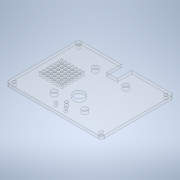
# Autodesk Inventor part: x_axis_plate_top_t
Saved by Autodesk Inventor 2022 (Build 260153000, 153)
## iProperties
Created: 2021-04-16
Part Number: x_axis_plate_top_t
Material: PET Plastic
Document SubType Name: Modeling
Designer: Fabijan_Sven
Density: 1.541 g/cm^3
Appearance: Polycarbonate - Clear
Mass: 164.884 g
Surface Area: 477.118 cm^2
Volume: 106.998 cm^3
Author: Fabijan_Sven
Autodesk Inventor part; units mm, degrees
ref_plane "YZ Plane" through (0, 0, 0) normal (1, 0, 0) x (0, 1, 0)
ref_plane "XZ Plane" through (0, 0, 0) normal (0, 1, 0) x (-1, 0, 0)
ref_plane "XY Plane" through (0, 0, 0) normal (0, 0, 1) x (1, 0, 0)
sketch "Sketch1" plane through (0, 0, 0) normal (0, 1, 0) x (-1, 0, 0)
  line L0 (-81, 62) -> (81, 62)
  line L1 (81, 62) -> (81, -62)
  line L2 (81, -62) -> (-81, -62)
  line L3 (-81, -62) -> (-81, 62)
  point P0 (0, 0)
  dimension "d117" = 124
  dimension "d118" = 162
  dimension "d119" = 81
  dimension "d120" = 62
  constraints: 8 end point, 2 parallel, 1 horizontal, 1 perpendicular
  measures "d117" distance between parallel lines of L2 L0
  measures "d118" distance between parallel lines of L1 L3
  measures "d119" distance from line of point (0, 0) L1
  measures "d120" distance from line of L2 point (0, 0)
extrude "Extrusion1" add sketch "Sketch1" along normal blind 5
fillet "Fillet1" radius 5 4 edges at (81, 2.5, 62) (81, 2.5, -62) (-81, 2.5, -62) (-81, 2.5, 62)
sketch "Sketch3" plane through (0, 5, 0) normal (0, 1, 0) x (1, 0, 0)
  circle A0 centre (74, -55) radius 3
  circle A1 centre (-74, -55) radius 3
  circle A2 centre (-74, 55) radius 3
  circle A3 centre (74, 55) radius 3
  line L0 (-76, -62) -> (76, -62) projected
  line L1 (81, -57) -> (81, 57) projected
  line L2 (-81, 57) -> (-81, -57) projected
  line L3 (76, 62) -> (-76, 62) projected
  point P0 (0, 0)
  dimension "d121" = 6
  dimension "d122" = 7
  dimension "d123" = 7
  dimension "d124" = 7
  dimension "d125" = 7
  constraints: 4 centre point, 3 equal radius, 2 horizontal alignment, 2 vertical alignment
  measures "d121" diameter of A0
  measures "d122" distance from line of L0 A0.centre
  measures "d123" distance from line of L1 A0.centre
  measures "d124" distance from line of L2 A1.centre
  measures "d125" distance from line of L3 A3.centre
hole "Hole1" at (74, 5, 55) at (-74, 5, 55) at (74, 5, -55) at (-74, 5, -55) direction (0, -1, 0) diameter 6 end through all
sketch "Sketch4" plane through (0, 5, 0) normal (0, 1, 0) x (1, 0, 0)
  circle A0 centre (26.1863, -35) radius 5
  circle A1 centre (-26.1863, -35) radius 5
  circle A2 centre (0, 10.5) radius 5
  circle A3 centre (26.1863, 35) radius 5
  circle A4 centre (-26.1863, 35) radius 5
  point P0 (0, 0)
  dimension "d130" = 10
  dimension "d131" = 24.5
  dimension "d132" = 70
  dimension "d133" = 52.3726
  dimension "d134" = 26.1863
  dimension "d135" = 26.1863
  dimension "d136" = 35
  constraints: 5 centre point, 4 equal radius, 2 horizontal alignment, 2 vertical alignment
  measures "d130" diameter of A1
  measures "d131" vertical distance of A4.centre A2.centre
  measures "d132" distance of A1.centre A4.centre
  measures "d133" distance of A1.centre A0.centre
  measures "d134" horizontal distance of A2.centre A4.centre
  measures "d135" horizontal distance of point (0, 0) A1.centre
  measures "d136" vertical distance of point (0, 0) A1.centre
hole "Hole2" at (-26.1863, 5, 35) at (26.1863, 5, 35) at (26.1863, 5, -35) at (-26.1863, 5, -35) direction (0, -1, 0) diameter 10 end through all
sketch "Sketch5" plane through (0, 0, 0) normal (0, -1, 0) x (1, 0, 0)
  circle A0 centre (0, 18.5) radius 9
  line L0 (-76, 62) -> (76, 62) projected
  point P0 (0, 0)
  dimension "d33" = 18
  dimension "d137" = 43.5
  constraints: 1 centre point, 1 vertical alignment
  measures "d33" diameter of A0
  measures "d137" distance from line of A0.centre L0
extrude "Extrusion3" cut sketch "Sketch5" against normal blind 10
sketch "Sketch7" plane through (0, 5, 0) normal (0, 1, 0) x (1, 0, 0)
  line L0 (9, 37) -> (-9, 37)
  line L1 (-9, 37) -> (-9, 72)
  line L2 (-9, 72) -> (9, 72)
  line L3 (9, 72) -> (9, 37)
  line L4 (76, 62) -> (-76, 62) projected
  point P0 (0, 0)
  point P1 (9, 62)
  point P2 (-9, 62)
  dimension "d138" = 35
  dimension "d139" = 10
  dimension "d140" = 18
  dimension "d141" = 9
  constraints: 8 end point, 2 parallel, 1 horizontal, 1 perpendicular
  measures "d138" distance between parallel lines of L2 L0
  measures "d139" distance between parallel lines of L4 L2
  measures "d140" distance between parallel lines of L3 L1
  measures "d141" distance from line of point (0, 0) L3
extrude "Extrusion5" cut sketch "Sketch7" against normal through all contours L0 L1 L4 L3
sketch "Sketch9" plane through (0, 5, 0) normal (0, 1, 0) x (1, 0, 0)
  circle A0 centre (-8.5, -49.5) radius 1.5
  circle A1 centre (8.5, -49.5) radius 1.5
  line L0 (-76, -62) -> (76, -62) projected
  line L1 (81, -57) -> (81, 57) projected
  line L2 (-81, 57) -> (-81, -57) projected
  dimension "d51" = 3
  dimension "d53" = 3
  dimension "d142" = 12.5
  dimension "d143" = 72.5
  dimension "d144" = 72.5
  constraints: 2 centre point, 1 horizontal alignment
  measures "d51" diameter of A1
  measures "d53" diameter of A0
  measures "d142" distance from line of L0 A1.centre
  measures "d143" distance from line of L1 A1.centre
  measures "d144" distance from line of L2 A0.centre
hole "Hole4" at (-8.5, 5, 49.5) at (8.5, 5, 49.5) direction (0, -1, 0) diameter 5 end through all
sketch "Sketch10" plane through (0, 5, 0) normal (0, 1, 0) x (1, 0, 0)
  circle A0 centre (0, -40) radius 3
  line L0 (-76, -62) -> (76, -62) projected
  point P0 (0, 0)
  dimension "d64" = 6
  dimension "d145" = 22
  constraints: 1 centre point, 1 vertical alignment
  measures "d64" diameter of A0
  measures "d145" distance from line of A0.centre L0
hole "Hole5" at (0, 5, 40) direction (0, -1, 0) diameter 6 depth 20 tip angle 118
sketch "Sketch13" plane through (0, 5, 0) normal (0, 1, 0) x (1, 0, 0)
  circle A0 centre (-66, 18) radius 2
  line L0 (-92, 62) -> (-157, 62) construction
  line L1 (-81, 110) -> (-81, -20) construction
  circle A1 centre (-66, 12) radius 2
  circle A2 centre (-66, 6) radius 2
  circle A3 centre (-66, 0) radius 2
  circle A4 centre (-66, -6) radius 2
  circle A5 centre (-66, -12) radius 2
  circle A6 centre (-66, -18) radius 2
  circle A7 centre (-60, 18) radius 2
  circle A8 centre (-60, 12) radius 2
  circle A9 centre (-60, 6) radius 2
  circle A10 centre (-60, 0) radius 2
  circle A11 centre (-60, -6) radius 2
  circle A12 centre (-60, -12) radius 2
  circle A13 centre (-60, -18) radius 2
  circle A14 centre (-54, 18) radius 2
  circle A15 centre (-54, 12) radius 2
  circle A16 centre (-54, 6) radius 2
  circle A17 centre (-54, 0) radius 2
  circle A18 centre (-54, -6) radius 2
  circle A19 centre (-54, -12) radius 2
  circle A20 centre (-54, -18) radius 2
  circle A21 centre (-48, 18) radius 2
  circle A22 centre (-48, 12) radius 2
  circle A23 centre (-48, 6) radius 2
  circle A24 centre (-48, 0) radius 2
  circle A25 centre (-48, -6) radius 2
  circle A26 centre (-48, -12) radius 2
  circle A27 centre (-48, -18) radius 2
  circle A28 centre (-42, 18) radius 2
  circle A29 centre (-42, 12) radius 2
  circle A30 centre (-42, 6) radius 2
  circle A31 centre (-42, 0) radius 2
  circle A32 centre (-42, -6) radius 2
  circle A33 centre (-42, -12) radius 2
  circle A34 centre (-42, -18) radius 2
  circle A35 centre (-36, 18) radius 2
  circle A36 centre (-36, 12) radius 2
  circle A37 centre (-36, 6) radius 2
  circle A38 centre (-36, 0) radius 2
  circle A39 centre (-36, -6) radius 2
  circle A40 centre (-36, -12) radius 2
  circle A41 centre (-36, -18) radius 2
  circle A42 centre (-30, 18) radius 2
  circle A43 centre (-30, 12) radius 2
  circle A44 centre (-30, 6) radius 2
  circle A45 centre (-30, 0) radius 2
  circle A46 centre (-30, -6) radius 2
  circle A47 centre (-30, -12) radius 2
  circle A48 centre (-30, -18) radius 2
  line L2 (-81, 57) -> (-81, -57) projected
  line L3 (-9, 62) -> (-76, 62) projected
  point P0 (0, 0)
  dimension "d101" = 44
  dimension "d102" = 15
  dimension "d103" = 4
  dimension "d106" = 6
  dimension "d109" = 6
  dimension "d146" = 0
  dimension "d147" = 0
  constraints: 49 centre point, 4 end point, 1 horizontal, 1 vertical, 96 other
  measures "d101" distance from line of L0 A0.centre
  measures "d102" distance from line of L1 A0.centre
  measures "d103" diameter of A0
  measures "d106" distance of A0.centre A1.centre
  measures "d109" distance of A0.centre A7.centre
  measures "d146" distance between parallel lines of L2 L1
  measures "d147" distance between parallel lines of L3 L0
extrude "Extrusion7" cut sketch "Sketch13" against normal through all
equation "\"d119\" = 0.5 * d118"
equation "\"d135\" = 0.5 * d133"
equation "\"d136\" = 0.5 * d132"
equation "\"d141\" = 0.5 * d140"
equation "\"d68\" = d64"
body "Solid1"
